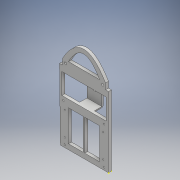
# Autodesk Inventor part: Base
Saved by Autodesk Inventor 2017 SP1 (Build 210196100, 196)
## iProperties
Part Number: Base
Material: Genérico
Document SubType Name: Modeling
Designer: Juan
Density: 1 g/cm^3
Appearance: Valor por defecto
Author: Juan
Autodesk Inventor part; units mm, degrees
ref_plane "YZ Plane" through (0, 0, 0) normal (1, 0, 0) x (0, 1, 0)
ref_plane "XZ Plane" through (0, 0, 0) normal (0, 1, 0) x (-1, 0, 0)
ref_plane "XY Plane" through (0, 0, 0) normal (0, 0, 1) x (1, 0, 0)
sketch "Boceto1" plane through (0, 0, 0) normal (0, 1, 0) x (-1, 0, 0)
  line L0 (0, 0) -> (0, 95)
  line L1 (0, 0) -> (65, 0)
  line L2 (65, 95) -> (66, 95)
  line L3 (66, 95) -> (62, 95)
  line L4 (0, 95) -> (4, 95)
  line L5 (66, 95) -> (4, 95)
  line L6 (66, 95) -> (54, 95) construction
  line L7 (54, 95) -> (54, 0)
  line L8 (0, 0) -> (12, 0) construction
  line L9 (12, 0) -> (12, 95)
  line L10 (54, 0) -> (34, 0) construction
  line L11 (34, 0) -> (54, 0) construction
  line L12 (12, 0) -> (32, 0) construction
  line L13 (54, 0) -> (54, 7)
  line L14 (54, 7) -> (12, 7)
  line L15 (34, 7) -> (34, 49)
  line L16 (34, 49) -> (54, 49)
  line L17 (32, 7) -> (32, 49)
  line L18 (32, 49) -> (12, 49)
  line L19 (54, 95) -> (54, 87) construction
  line L20 (54, 87) -> (12, 87)
  line L21 (54, 49) -> (54, 59) construction
  line L22 (54, 59) -> (12, 59)
  line L23 (66, 95) -> (65, 0)
  line L24 (4, 95) -> (4, 103)
  line L25 (4, 103) -> (62, 103)
  line L26 (62, 103) -> (62, 95)
  line L27 (4, 103) -> (34, 152.6106) construction
  line L28 (34, 152.6106) -> (62, 103) construction
  spline S0 degree 2 poles (4, 103) (34, 152.6106) (62, 103) knots 1 1 1 2 2 2
  line L29 (4, 103) -> (12, 103) construction
  line L30 (62, 103) -> (54, 103) construction
  line L31 (54, 103) -> (34, 141.3072) construction
  line L32 (34, 141.3072) -> (12, 103) construction
  spline S1 degree 2 poles (54, 103) (34, 141.3072) (12, 103) knots 1 1 1 2 2 2
  line L33 (62, 99) -> (4, 99) construction
  line L34 (8, 95) -> (8, 103) construction
  line L35 (58.1768, 95) -> (58.1768, 103) construction
  circle A0 centre (8, 99) radius 1.5
  circle A1 centre (58.1768, 99) radius 1.5
  dimension "d0" = 95
  dimension "d3" = 4
  dimension "d4" = 4
  dimension "d14" = 12
  dimension "d19" = 42
  dimension "d20" = 8
  dimension "d22" = 42
  dimension "d23" = 42
  dimension "d24" = 20
  dimension "d25" = 20
  dimension "d27" = 62
  dimension "d37" = 65
  dimension "d38" = 89.397
  dimension "d41" = 46
  dimension "d42" = 36
  dimension "d43" = 0.9999
  dimension "d44" = 30.9983
  dimension "d45" = 32.9982
  dimension "d76" = 8
  dimension "d77" = 8
  dimension "d78" = 8
  dimension "d79" = 60.56
  dimension "d80" = 117.569
  dimension "d81" = 60.131
  dimension "d82" = 58.838
  dimension "d83" = 24.1768
  dimension "d84" = 3
  dimension "d85" = 3
  constraints: 64 end point, 24 point on line, 11 perpendicular, 5 midpoint, 3 parallel, 2 centre point, 2 vertical, 1 collinear, 6 other
  measures "d0" distance of L0.start L0.end
  measures "d3" distance of L2.end L3.end
  measures "d4" distance of L0.end L4.end
  measures "d14" distance of L0.start L8.end
  measures "d19" distance of L15.start L15.end
  measures "d20" distance of L6.end L19.end
  measures "d22" distance of L21.end L22.end
  measures "d23" distance of L19.end L20.end
  measures "d24" distance of L17.end L18.end
  measures "d25" distance of L15.end L16.end
  measures "d27" distance of L2.end L4.end
  measures "d37" distance of L0.start L1.end
  measures "d38" angle of L6 L23
  measures "d41" distance between parallel lines of L3 L16
  measures "d42" distance between parallel lines of L3 L22
  measures "d43" distance from line of L2.start L23
  measures "d44" distance from line of L10.end L23
  measures "d45" distance from line of L12.end L23
  measures "d76" distance of L4.end L24.end
  measures "d77" distance of L24.end L29.end
  measures "d78" distance of L25.end L30.end
  measures "d79" angle of L28 L2
  measures "d80" angle of L31 L2
  measures "d81" angle of L32 L2
  measures "d82" angle of L27 L2
  measures "d83" distance between parallel lines of L35 L15
  measures "d84" diameter of A0
  measures "d85" diameter of A1
extrude "Extrusión1" add sketch "Boceto1" along normal blind 4 contours L0 L4 L5 L9 L1 | L9 L14 L7 L1 | L24 L25 L26 L5 | L7 L5 L3 L2 L23 L1 | L5 L7 L20 L9 | S0 L25 S1 | L9 L22 L7 L16 L15 L14 L17 L18 | A0 | A1
ref_plane "Plano de trabajo1" through (0, 4, 0) normal (0, 1, 0) x (1, 0, 0)
sketch "Boceto2" plane through (0, 4, 0) normal (0, 1, 0) x (1, 0, 0)
  line L0 (-54, -59) -> (-12, -59) projected
  line L1 (-12, -59) -> (-12, -87) projected
  line L2 (-12, -87) -> (-54, -87) projected
  line L3 (-54, -87) -> (-54, -59) projected
  line L4 (-54, -49) -> (-54, -7) projected
  line L5 (-54, -7) -> (-34, -7) projected
  line L6 (-34, -7) -> (-34, -49) projected
  line L7 (-34, -49) -> (-54, -49) projected
  line L8 (-4, -95) -> (0, -95) projected
  line L9 (-12, -49) -> (-32, -49) projected
  line L10 (-32, -49) -> (-32, -7) projected
  line L11 (-32, -7) -> (-12, -7) projected
  line L12 (-12, -7) -> (-12, -49) projected
  line L13 (0, 0) -> (-65, 0) projected
  line L14 (-65, 0) -> (-66, -95) projected
  line L15 (0, -95) -> (0, 0) projected
  line L16 (-54, -59) -> (-12, -59) projected
  line L17 (0, 0) -> (-65, 0) construction
  line L18 (0, -95) -> (0, 0) construction
  circle A0 centre (-5.9989, -3.4994) radius 2.5
  circle A1 centre (-59.0011, -3.4994) radius 2.5
  line L19 (-12, -49) -> (-32, -49) construction
  circle A2 centre (-6, -54) radius 2.5
  circle A3 centre (-61, -54) radius 2.5
  line L20 (-66, -95) -> (-62, -95) projected
  line L21 (-62, -95) -> (-62, -103) projected
  line L22 (-54, -103) -> (-12, -103) projected
  line L23 (-4, -103) -> (-4, -95) projected
  line L24 (-62, -99) -> (-4, -99) construction
  line L25 (-4, -103) -> (-4, -95) construction
  dimension "d54" = 5
  dimension "d58" = 5
  dimension "d60" = 5
  dimension "d61" = 3.4994
  dimension "d62" = 5.9989
  dimension "d63" = 54
  dimension "d64" = 6
  dimension "d65" = 3.4994
  dimension "d66" = 59.0011
  dimension "d67" = 54
  dimension "d68" = 61
  constraints: 4 centre point, 2 end point, 2 horizontal alignment, 2 midpoint, 1 equal radius
  measures "d54" diameter of A0
  measures "d58" diameter of A2
  measures "d60" diameter of A3
  measures "d61" distance from line of A0.centre L13
  measures "d62" distance from line of A0.centre L15
  measures "d63" distance from line of A2.centre L13
  measures "d64" distance from line of A2.centre L15
  measures "d65" distance from line of A1.centre L13
  measures "d66" distance from line of A1.centre L15
  measures "d67" distance from line of A3.centre L13
  measures "d68" distance from line of A3.centre L15
hole "Agujero1" at (-6, 4, 54) at (-61, 4, 54) at (-59.0011, 4, 3.4994) at (-5.9989, 4, 3.4994) direction (0, -1, 0) diameter 2.057 end through all
sketch "Boceto3" plane through (0, 4, 0) normal (0, 1, 0) x (1, 0, 0)
  point P0 (0, 0)
sketch "Boceto4" plane through (0, 0, 0) normal (0, -1, 0) x (1, 0, 0)
  point P0 (0, 0)
ref_plane "Plano de trabajo2" through (0, 0, 0) normal (0, -1, 0) x (1, 0, 0)
sketch "Boceto6" plane through (0, 0, 0) normal (0, -1, 0) x (1, 0, 0)
  point P0 (0, 0)
sketch "Boceto7" plane through (0, 0, 0) normal (0, -1, 0) x (1, 0, 0)
  point P0 (0, 0)
ref_plane "Plano de trabajo3" through (0, 0, 0) normal (0, -1, 0) x (1, 0, 0)
sketch "Boceto8" plane through (0, 0, 0) normal (0, -1, 0) x (1, 0, 0)
  point P0 (0, 0)
sketch "Boceto9" plane through (0, 0, 0) normal (0, -1, 0) x (1, 0, 0)
  line L0 (-62, 95) -> (-62, 103) construction
  line L1 (-62, 103) -> (-62, 99) construction
  line L2 (-62, 99) -> (-58.0035, 99) construction
  line L3 (-4, 95) -> (0, 95) construction
  line L4 (-4, 95) -> (-4, 99) construction
  line L5 (-4, 103) -> (-4, 95) construction
  line L6 (-4, 99) -> (-7.9965, 99) construction
  point P0 (0, 0)
  dimension "d116" = 4
  dimension "d117" = 3.9965
  dimension "d118" = 4
  dimension "d119" = 3.9965
  constraints: 8 end point, 2 midpoint, 2 perpendicular
  measures "d116" distance of L0.end L1.end
  measures "d117" distance of L1.end L2.end
  measures "d118" distance of L3.start L4.end
  measures "d119" distance of L4.end L6.end
hole "Agujero5" at (-58.0035, 0, 99.0001) direction (0, 1, 0) diameter 3 end through all
hole "Agujero6" at (-7.9965, 0, 99) direction (0, 1, 0) diameter 3 end through all
ref_plane "Plano de trabajo4" through (0, 2, 0) normal (0, 1, 0) x (1, 0, 0)
sketch "Boceto11" plane through (0, 4, 0) normal (0, 1, 0) x (1, 0, 0)
  line L0 (-32, -7) -> (-12, -7) construction
  line L1 (-12, -7) -> (-12, -12) construction
  line L2 (-12, -7) -> (-12, -49) construction
  line L3 (-12, -12) -> (-7, -12) construction
  line L4 (-12, -49) -> (-12, -44) construction
  line L5 (-54, -7) -> (-34, -7) construction
  line L6 (-54, -7) -> (-54, -12) construction
  line L7 (-54, -49) -> (-54, -7) construction
  line L8 (-54, -12) -> (-59, -12) construction
  line L9 (-12, -44) -> (-7, -44) construction
  line L10 (-54, -49) -> (-54, -44) construction
  line L11 (-54, -44) -> (-59, -44) construction
  point P0 (0, 0)
  dimension "d150" = 5
  dimension "d151" = 5
  dimension "d152" = 5
  dimension "d153" = 5
  dimension "d154" = 5
  dimension "d155" = 5
  constraints: 16 end point, 4 point on line, 3 horizontal, 1 perpendicular
  measures "d150" distance of L0.end L1.end
  measures "d151" distance of L1.end L3.end
  measures "d152" distance of L2.end L4.end
  measures "d153" distance of L5.start L6.end
  measures "d154" distance of L6.end L8.end
  measures "d155" distance of L7.start L10.end
hole "Agujero8" at (-7, 4, 12) at (-7, 4, 44) at (-59, 4, 12) at (-59, 4, 44) direction (0, -1, 0) diameter 1.778 end through all
sketch "Boceto12" plane through (0, 4, 0) normal (0, 1, 0) x (1, 0, 0)
  line L0 (-43, -59) -> (-43, -58) construction
  line L1 (-23, -87) -> (-43, -87) construction
  line L2 (-43, -87) -> (-43, -88.5) construction
  line L3 (-43, -88.5) -> (-23, -88.5) construction
  line L4 (-23, -88.5) -> (-23, -87) construction
  line L5 (-23, -59) -> (-43, -59) construction
  line L6 (-43, -59) -> (-43, -57.5) construction
  line L7 (-43, -57.5) -> (-23, -57.5) construction
  line L8 (-23, -57.5) -> (-23, -59) construction
  line L9 (-23, -59) -> (-43, -59)
  line L10 (-43, -59) -> (-43, -57.5)
  line L11 (-43, -57.5) -> (-23, -57.5)
  line L12 (-23, -57.5) -> (-23, -59)
  line L13 (-23, -87) -> (-43, -87)
  line L14 (-43, -87) -> (-43, -88.5)
  line L15 (-43, -88.5) -> (-23, -88.5)
  line L16 (-23, -88.5) -> (-23, -87)
  point P0 (0, 0)
  point P1 (-12, -59)
  dimension "d168" = 1.5
  constraints: 34 end point, 8 parallel, 4 horizontal, 4 perpendicular
  measures "d168" distance of L2.end L1.end
extrude "Extrusión2" add sketch "Boceto12" along normal blind 12
sketch "Boceto14" plane through (-12, 0, 87) normal (0, 0, -1) x (-1, 0, 0)
  line L0 (11, 16) -> (31, 16) projected
  line L1 (31, 4) -> (31, 16) projected
  line L2 (11, 16) -> (31, 16)
  line L3 (31, 16) -> (31, 14)
  line L4 (31, 14) -> (11, 14)
  line L5 (11, 14) -> (11, 16)
  point P0 (-12, 0)
  dimension "d173" = 2
  constraints: 8 end point, 2 parallel, 1 horizontal, 1 perpendicular, 1 point on line
  measures "d173" distance of L2.end L3.end
extrude "Extrusión3" add sketch "Boceto14" along normal blind 28
ref_plane "Plano de trabajo7" through (0, 16, 0) normal (0, 1, 0) x (1, 0, 0)
sketch "Boceto15" plane through (0, 16, 0) normal (0, 1, 0) x (1, 0, 0)
  line L0 (-43, -57.5) -> (-23, -57.5) construction
  line L1 (-23, -88.5) -> (-43, -88.5) construction
  line L2 (-23, -57.5) -> (-43, -88.5) construction
  line L3 (-23, -88.5) -> (-43, -57.5) construction
  line L4 (-33, -73) -> (-23, -73) construction
  line L5 (-23, -88.5) -> (-23, -57.5) construction
  point P0 (0, 0)
  constraints: 6 end point, 2 midpoint
hole "Agujero9" at (-33, 16, 73) direction (0, -1, 0) diameter 3 depth 8 tip angle 118
fillet "Empalme1" radius 3 2 edges at (-33, 16, 57.5) (-33, 16, 88.5)
sketch "Boceto16" plane through (-54, 0, 87) normal (1, 0, 0) x (0, 0, -1)
  line L0 (0, 4) -> (28, 4)
  line L1 (28, 4) -> (28, 0)
  line L2 (28, 0) -> (0, 0)
  line L3 (0, 0) -> (0, 4)
  point P0 (87, 0)
  constraints: 8 end point, 2 parallel, 1 horizontal, 1 perpendicular
extrude "Extrusión4" cut sketch "Boceto16" against normal blind 9
sketch "Boceto17" plane through (-12, 0, 59) normal (-1, 0, 0) x (0, 0, 1)
  line L0 (0, 0) -> (0, 4) projected
  line L1 (0, 0) -> (28, 0) projected
  line L2 (0, 4) -> (28, 4)
  line L3 (28, 4) -> (28, 0)
  line L4 (28, 0) -> (0, 0)
  line L5 (0, 0) -> (0, 4)
  point P0 (-59, 0)
  constraints: 8 end point, 2 parallel, 1 horizontal, 1 perpendicular
extrude "Extrusión5" cut sketch "Boceto17" against normal blind 9
